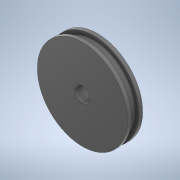
# Autodesk Inventor part: AM_Pulley
Saved by Autodesk Inventor 2020.1 (Build 241239000, 239)
## iProperties
Created: 2019-12-04
Part Number: AM_Pulley
Material: ABS Plastic
Document SubType Name: Modeling
Designer: tbloo
Density: 1.06 g/cm^3
Appearance: Smooth - Black
Author: tbloo
Autodesk Inventor part; units mm, degrees
ref_plane "YZ Plane" through (0, 0, 0) normal (1, 0, 0) x (0, 1, 0)
ref_plane "XZ Plane" through (0, 0, 0) normal (0, 1, 0) x (-1, 0, 0)
ref_plane "XY Plane" through (0, 0, 0) normal (0, 0, 1) x (1, 0, 0)
sketch "Sketch1" plane through (0, 0, 0) normal (1, 0, 0) x (0, 1, 0)
  line L0 (7.1438, 2.3813) -> (7.9375, 2.3813)
  line L1 (7.9375, 1.5875) -> (7.935, 1.5875)
  line L2 (7.935, 0.8096) -> (7.9375, 0.8096)
  line L3 (7.1438, 0.7937) -> (7.9375, 0.795)
  line L4 (7.1438, 2.3813) -> (7.1438, 0.7937)
  line L5 (7.9375, 3.175) -> (7.9375, 2.3813)
  line L6 (7.9375, 0.795) -> (7.9375, 0)
  line L7 (-1.5875, 3.175) -> (-1.5875, 0)
  line L8 (0, 3.175) -> (0, 0)
  line L9 (-1.5875, 0) -> (-1.5875, 3.175)
  line L10 (0, 3.175) -> (7.9375, 3.175)
  line L11 (7.9375, 0) -> (0, 0)
  point P0 (0, 0)
  dimension "d1" = 3.175
  dimension "d2" = 0.7937
  dimension "d4" = 0.0025
  dimension "d5" = 0.7937
  dimension "d9" = 9.525
  dimension "d10" = 1.5875
  constraints: 24 end point, 3 parallel, 2 horizontal, 2 vertical, 1 collinear
  measures "d1" distance of L5.start L6.end
  measures "d2" distance of L0.start L0.end
  measures "d4" distance of L2.end L2.start
  measures "d5" distance of L3.end L3.start
  measures "d9" distance of L5.start L7.start
  measures "d10" distance of L8.end L9.start
revolve "Revolution2" add sketch "Sketch1" angle 360 about axis through (0, -1.5875, 0) along (0, 0, 1)
body "Solid2"
